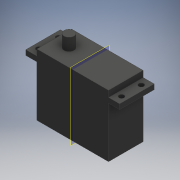
# Autodesk Inventor part: Shoulder Servo
Saved by Autodesk Inventor 2017 (Build 210142000, 142)
## iProperties
Created: 2018-10-14
Part Number: Shoulder Servo
Material: Generic
Document SubType Name: Modeling
Designer: Cameron
Density: 1 g/cm^3
Appearance: Generic
Author: Cameron
Autodesk Inventor part; units mm, degrees
ref_plane "YZ Plane" through (0, 0, 0) normal (1, 0, 0) x (0, 1, 0)
ref_plane "XZ Plane" through (0, 0, 0) normal (0, 1, 0) x (-1, 0, 0)
ref_plane "XY Plane" through (0, 0, 0) normal (0, 0, 1) x (1, 0, 0)
sketch "Sketch1" plane through (0, 0, 0) normal (0, 0, 1) x (1, 0, 0)
  line L0 (0, 0) -> (58, 0)
  line L1 (58, 0) -> (58, 28)
  line L2 (58, 28) -> (0, 28)
  line L3 (0, 28) -> (0, 0)
  dimension "d0" = 58
  dimension "d1" = 28
  constraints: 8 end point, 2 parallel, 1 horizontal, 1 perpendicular
  measures "d0" distance of L2.end L1.end
  measures "d1" distance of L1.end L0.end
extrude "Extrusion1" add sketch "Sketch1" along normal blind 50
sketch "Sketch2" plane through (58, 0, 0) normal (1, 0, 0) x (0, 0, -1)
  line L0 (0, 28) -> (-50, 28) projected
  line L1 (0, 0) -> (-50, 0) projected
  line L2 (-50, 28) -> (-45, 28)
  line L3 (-45, 28) -> (-45, 0)
  line L4 (-45, 28) -> (-41, 28)
  line L5 (-41, 28) -> (-41, 0)
  line L6 (-41, 0) -> (-45, 0)
  line L7 (-45, 0) -> (-45, 28)
  dimension "d4" = 5
  dimension "d5" = 4
  constraints: 12 end point, 3 point on line, 2 parallel, 2 perpendicular, 1 horizontal
  measures "d4" distance of L0.end L2.end
  measures "d5" distance of L5.end L6.end
extrude "Extrusion2" add sketch "Sketch2" along normal blind 9
ref_plane "Work Plane1" through (29, 0, 0) normal (-1, 0, 0) x (0, 0, 1)
mirror "Mirror1" about plane through (29, 0, 0) normal (-1, 0, 0) of "Extrusion2"
sketch "Sketch3" plane through (-9, 28, 45) normal (0, 0, 1) x (1, 0, 0)
  line L0 (9, 0) -> (0, 0) projected
  line L1 (4.5, 0) -> (4.5, -6)
  line L2 (9, -28) -> (0, -28) projected
  line L3 (4.5, -6) -> (4.5, -22)
  circle A0 centre (4.5, -6) radius 2
  circle A1 centre (4.5, -22) radius 2
  dimension "d8" = 6
  dimension "d9" = 16
  dimension "d10" = 4
  dimension "d11" = 4
  constraints: 4 end point, 2 centre point, 2 coincident, 1 midpoint, 1 perpendicular, 1 point on line
  measures "d8" distance of L1.start L1.end
  measures "d9" distance of L1.end L3.end
  measures "d10" diameter of A0
  measures "d11" diameter of A1
extrude "Extrusion3" cut sketch "Sketch3" against normal blind 9
sketch "Sketch4" plane through (58, 0, 45) normal (0, 0, 1) x (1, 0, 0)
  circle A0 centre (-62.5, 22) radius 2 projected
  line L0 (-62.5, 22) -> (4.5, 22)
  line L1 (4.5, 22) -> (4.5, 6)
  circle A1 centre (4.5, 22) radius 2
  circle A2 centre (4.5, 6) radius 2
  point P0 (-58, 0)
  dimension "d14" = 16
  dimension "d15" = 4
  dimension "d16" = 4
  constraints: 4 end point, 2 centre point, 2 coincident, 1 horizontal, 1 perpendicular
  measures "d14" distance of L0.end L1.end
  measures "d15" diameter of A1
  measures "d16" diameter of A2
extrude "Extrusion4" cut sketch "Sketch4" against normal blind 9 contours A1 L1 L0 | L0 L1 A1 | A2
sketch "Sketch5" plane through (0, 0, 50) normal (0, 0, 1) x (1, 0, 0)
  line L0 (0, 28) -> (0, 0) projected
  line L1 (0, 14) -> (12, 14)
  circle A0 centre (12, 14) radius 4
  dimension "d19" = 12
  dimension "d20" = 8
  constraints: 2 end point, 1 centre point, 1 coincident, 1 horizontal, 1 midpoint
  measures "d19" distance of L1.start L1.end
  measures "d20" diameter of A0
extrude "Extrusion5" add sketch "Sketch5" along normal blind 10
body "Solid1"
